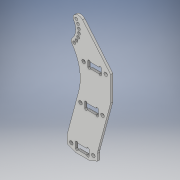
# Autodesk Inventor part: 頭＿メインフレーム
Saved by Autodesk Inventor 2018 (Build 220112000, 112)
## iProperties
Created: 2018-06-07
Part Number: 頭＿メインフレーム
Material: 一般
Document SubType Name: Modeling
Designer: taka
Density: 1 g/cm^3
Appearance: 既定
Author: taka
Autodesk Inventor part; units mm, degrees
ref_plane "YZ Plane" through (0, 0, 0) normal (1, 0, 0) x (0, 1, 0)
ref_plane "XZ Plane" through (0, 0, 0) normal (0, 1, 0) x (-1, 0, 0)
ref_plane "XY Plane" through (0, 0, 0) normal (0, 0, 1) x (1, 0, 0)
sketch "スケッチ1" plane through (0, 0, 0) normal (0, 1, 0) x (-1, 0, 0)
  line L0 (0, 0) -> (7, 0)
  line L1 (7, 0) -> (7, -27) construction
  line L2 (7, -27) -> (0, -27)
  line L3 (0, -27) -> (0, 0) construction
  circle A0 centre (2.5, -3.7) radius 1.6
  circle A1 centre (2.5, -23.3) radius 1.6
  line L4 (5.05, -7.5) -> (0.05, -7.5) construction
  line L5 (0.05, -7.5) -> (0.05, -19.5) construction
  line L6 (0.05, -19.5) -> (5.05, -19.5) construction
  line L7 (5.05, -19.5) -> (5.05, -7.5) construction
  line L8 (0, -7.45) -> (5.1, -7.45)
  line L9 (5.1, -7.45) -> (5.1, -19.55)
  line L10 (5.1, -19.55) -> (0, -19.55)
  line L11 (0, -19.55) -> (0, -7.45)
  line L12 (84.5459, 21.5815) -> (61.9185, -1.0459) construction
  line L13 (61.9185, -1.0459) -> (65.4541, -4.5815) construction
  line L14 (65.4541, -4.5815) -> (88.0815, 18.0459) construction
  line L15 (88.0815, 18.0459) -> (84.5459, 21.5815) construction
  line L16 (70.3953, 0.3598) -> (83.1317, 13.0962)
  circle A2 centre (100.1023, -8.117) radius 1.25
  line L17 (7, 0) -> (45.561, -10.3324)
  line L18 (7, -27) -> (50.4418, -38.6402)
  line L19 (72.4418, -38.6402) -> (106.1477, -10.3575)
  line L20 (106.1477, -10.3575) -> (100.2529, -4.1751)
  arc A3 (45.561, -10.3324) -> (81.4937, -2.447) centre (55.9138, 28.3046) ccw
  line L21 (72.4418, -38.6402) -> (50.4418, -38.6402)
  line L22 (40, -9.2) -> (35, -9.2) construction
  line L23 (35, -9.2) -> (35, -34.2) construction
  line L24 (35, -34.2) -> (40, -34.2) construction
  line L25 (40, -34.2) -> (40, -9.2) construction
  circle A4 centre (97.0056, -9.675) radius 1.25
  circle A5 centre (93.6401, -10.5063) radius 1.25
  circle A6 centre (90.1742, -10.5693) radius 1.25
  circle A7 centre (86.7807, -9.8609) radius 1.25
  circle A8 centre (83.6295, -8.4164) radius 1.25
  circle A9 centre (80.8777, -6.3081) radius 1.25
  line L26 (100.2529, -4.1751) -> (104.1748, -8.2883)
  arc A10 (81.4937, -2.447) -> (100.2529, -4.1751) centre (91.6271, 4.8718) ccw
  line L27 (40, -15.7) -> (35, -15.7) construction
  line L28 (35, -15.7) -> (35, -27.7) construction
  line L29 (35, -27.7) -> (40, -27.7) construction
  line L30 (40, -27.7) -> (40, -15.7) construction
  line L31 (34.95, -15.65) -> (40.05, -15.65)
  line L32 (40.05, -15.65) -> (40.05, -27.75)
  line L33 (40.05, -27.75) -> (34.95, -27.75)
  line L34 (34.95, -27.75) -> (34.95, -15.65)
  circle A11 centre (37.5, -11.9) radius 1.6
  circle A12 centre (37.5, -31.5) radius 1.6
  line L35 (73, -12) -> (68, -12) construction
  line L36 (68, -12) -> (68, -37) construction
  line L37 (68, -37) -> (73, -37) construction
  line L38 (73, -37) -> (73, -12) construction
  line L39 (73, -18.5) -> (68, -18.5) construction
  line L40 (68, -18.5) -> (68, -30.5) construction
  line L41 (68, -30.5) -> (73, -30.5) construction
  line L42 (73, -30.5) -> (73, -18.5) construction
  line L43 (67.95, -18.45) -> (73.05, -18.45)
  line L44 (73.05, -18.45) -> (73.05, -30.55)
  line L45 (73.05, -30.55) -> (67.95, -30.55)
  line L46 (67.95, -30.55) -> (67.95, -18.45)
  circle A13 centre (70.5, -14.7) radius 1.6
  circle A14 centre (70.5, -34.3) radius 1.6
  circle A15 centre (73.05, -19.5) radius 1.05
  circle A16 centre (67.95, -19.5) radius 1.05
  circle A17 centre (67.95, -29.5) radius 1.05
  circle A18 centre (73.05, -29.5) radius 1.05
  circle A19 centre (40.05, -16.7) radius 1.05
  circle A20 centre (34.95, -16.7) radius 1.05
  circle A21 centre (34.95, -26.7) radius 1.05
  circle A22 centre (40.05, -26.7) radius 1.05
  circle A23 centre (5.1, -8.5) radius 1.05
  circle A24 centre (0, -8.5) radius 1.05
  circle A25 centre (0, -18.5) radius 1.05
  circle A26 centre (5.1, -18.5) radius 1.05
  line L47 (-3, -7.45) -> (-3, -19.55)
  line L48 (-3, -19.55) -> (0, -27)
  line L49 (-3, -7.45) -> (0, 0)
  circle A27 centre (91.6271, 4.8718) radius 15.5
  point P0 (75, 8.5)
  point P1 (91.6085, -20.8534)
  point P2 (82.042, -3.1517)
  point P3 (81.2596, -2.6403)
  point P4 (55.561, -0.3324)
  point P5 (40, -14.6)
  point P6 (35, -14.6)
  point P7 (40, -28.8)
  point P8 (35, -28.8)
  dimension "d0" = 7
  dimension "d1" = 27
  dimension "d2" = 3.2
  dimension "d3" = 3.2
  dimension "d4" = 5
  dimension "d5" = 12
  dimension "d6" = 2.5
  dimension "d7" = 2.5
  dimension "d8" = 19.6
  dimension "d9" = 3.7
  dimension "d11" = 7.5
  dimension "d12" = 0.05
  dimension "d20" = 32
  dimension "d21" = 5
  dimension "d22" = 45
  dimension "d23" = 2.5
  dimension "d24" = 16
  dimension "d25" = 75
  dimension "d26" = 8.5
  dimension "d27" = 30
  dimension "d33" = 27
  dimension "d35" = 2.5
  dimension "d44" = 75
  dimension "d49" = 75
  dimension "d52" = 40
  dimension "d53" = 30
  dimension "d56" = 39
  dimension "d61" = 5
  dimension "d62" = 25
  dimension "d63" = 33
  dimension "d64" = 9.2
  dimension "d69" = 77
  dimension "d72" = 22
  dimension "d73" = 12.5
  dimension "d74" = 50
  dimension "d75" = 21
  dimension "d76" = 44
  dimension "d77" = 12
  dimension "d78" = 6.5
  dimension "d79" = 0.05
  dimension "d84" = 3.2
  dimension "d85" = 2.5
  dimension "d86" = 2.7
  dimension "d88" = 3.2
  dimension "d89" = 19.6
  dimension "d90" = 2.5
  dimension "d91" = 5
  dimension "d92" = 25
  dimension "d93" = 12
  dimension "d94" = 6.5
  dimension "d95" = 0.05
  dimension "d100" = 3.2
  dimension "d101" = 2.5
  dimension "d102" = 2.7
  dimension "d104" = 3.2
  dimension "d105" = 19.6
  dimension "d106" = 2.5
  dimension "d107" = 12
  dimension "d109" = 66
  dimension "d118" = 2.1
  dimension "d119" = 2.1
  dimension "d120" = 2.1
  dimension "d121" = 2.1
  dimension "d122" = 2.1
  constraints: 100 end point, 28 centre point, 21 point on line, 20 parallel, 13 tangent, 10 perpendicular, 7 horizontal, 6 point on circle, 4 collinear, 3 coincident, 1 vertical, 22 other
  measures "d0" distance of L1.end L2.end
  measures "d1" distance of L0.end L1.end
  measures "d2" diameter of A0
  measures "d3" diameter of A1
  measures "d4" distance of L6.end L5.end
  measures "d5" distance of L5.end L4.end
  measures "d6" distance from line of L3 A0.centre
  measures "d7" distance from line of L3 A1.centre
  measures "d8" distance of A1.centre A0.centre
  measures "d9" vertical distance of L0.start A0.centre
  measures "d11" distance between parallel lines of L0 L4
  measures "d12" distance between parallel lines of L4 L8
  measures "d20" distance of L14.end L13.end
  measures "d21" distance of L13.end L12.end
  measures "d22" angle of L0 L14
  measures "d23" distance from line of point (75, 8.5) L14
  measures "d24" distance from line of L15 point (75, 8.5)
  measures "d25" distance from line of point (75, 8.5) L3
  measures "d26" distance from line of point (75, 8.5) L0
  measures "d27" distance of point (91.609, -20.853) L16.start
  measures "d33" distance from line of L14 point (100.102, -8.117)
  measures "d35" diameter of A2
  measures "d44" angle of L1 L17
  measures "d49" angle of L18 L1
  measures "d52" radius of A3
  measures "d53" distance from line of L16 A3.centre
  measures "d56" distance from line of L21 L16.start
  measures "d61" distance of L24.end L23.end
  measures "d62" distance of L23.end L22.end
  measures "d63" distance between parallel lines of L1 L25
  measures "d64" distance between parallel lines of L22 L0
  measures "d72" distance of L19.start L18.end
  measures "d73" radius of A10
  measures "d74" angle of L3 L19
  measures "d75" distance from line of point (91.627, 4.872) L19
  measures "d76" distance of L19.start L19.end
  measures "d77" distance of L28.end L27.end
  measures "d78" distance between parallel lines of L24 L29
  measures "d79" distance between parallel lines of L27 L31
  measures "d84" diameter of A11
  measures "d85" distance from line of L23 A11.centre
  measures "d86" distance from line of L22 A11.centre
  measures "d88" diameter of A12
  measures "d89" distance of A12.centre A11.centre
  measures "d90" distance from line of L23 A12.centre
  measures "d91" distance of L37.end L37.start
  measures "d92" distance of L37.start L36.start
  measures "d93" distance of L41.start L40.start
  measures "d94" distance between parallel lines of L37 L41
  measures "d95" distance between parallel lines of L39 L43
  measures "d100" diameter of A13
  measures "d101" distance from line of L36 A13.centre
  measures "d102" distance from line of L35 A13.centre
  measures "d104" diameter of A14
  measures "d105" distance of A14.centre A13.centre
  measures "d106" distance from line of L36 A14.centre
  measures "d107" distance between parallel lines of L0 L35
  measures "d109" distance between parallel lines of L1 L38
  measures "d118" diameter of A15
  measures "d119" diameter of A16
  measures "d120" diameter of A17
  measures "d121" diameter of A18
  measures "d122" diameter of A19
extrude "押し出し2" add sketch "スケッチ1" along normal blind 2 contours L0 L17 A3 A27 A9 A8 A7 A6 A5 A4 A2 L20 L19 L21 L18 L2 L48 L47 L49 | A3 A10 L20 A27 A2 A4 A5 A6 A7 A8 A9
fillet "フィレット1" radius 5 1 edges at (-106.1477, 1, -10.3575)
fillet "フィレット2" radius 3 2 edges at (-81.4937, 1, -2.447) (-100.2529, 1, -4.1751)
fillet "フィレット3" radius 8 2 edges at (-7, 1, -27) (-7, 1, 0)
equation "\"d7\" = d6"
equation "\"d11\" = -0.5 * d5 + 0.5 * d1"
equation "\"d23\" = 0.5 * d21"
equation "\"d24\" = 0.5 * d20"
equation "\"d49\" = d44"
equation "\"d28\" = d20 - 2 * d29"
equation "\"d29\" = 7"
